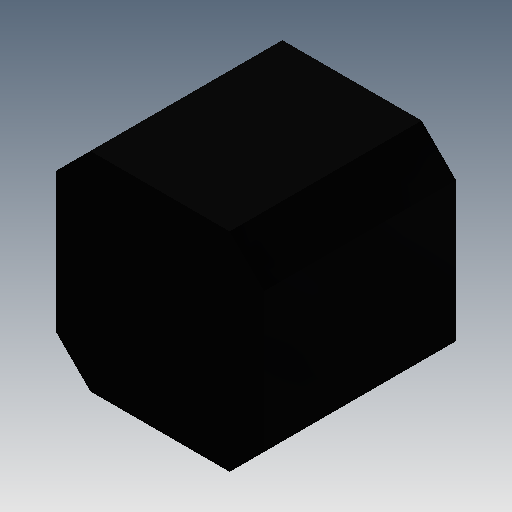
# Autodesk Inventor part: Nema 17 Body
Saved by Autodesk Inventor 2020.3 (Build 243373000, 373)
## iProperties
Created: 2015-09-21
Part Number: Nema 17 Body
Material: Aluminum 6061
Document SubType Name: Modeling
Designer: Dr Kreigar
Density: 2.7 g/cm^3
Appearance: Anodized - Black
Mass: 178.094 g
Surface Area: 93.4175 cm^2
Volume: 65.9607 cm^3
Author: Dr Kreigar
Autodesk Inventor part; units mm, degrees
ref_plane "YZ Plane" through (0, 0, 0) normal (1, 0, 0) x (0, 1, 0)
ref_plane "XZ Plane" through (0, 0, 0) normal (0, 1, 0) x (-1, 0, 0)
ref_plane "XY Plane" through (0, 0, 0) normal (0, 0, 1) x (1, 0, 0)
sketch "Sketch1" plane through (0, 0, 0) normal (0, 0, 1) x (1, 0, 0)
  line L0 (21.15, -14.1503) -> (21.15, 14.1503) construction
  line L1 (14.1503, 21.15) -> (21.15, 14.1503) construction
  line L2 (14.1503, 21.15) -> (-14.1503, 21.15) construction
  line L3 (-21.15, 14.1503) -> (-14.1503, 21.15) construction
  line L4 (-21.15, 14.1503) -> (-21.15, -14.1503) construction
  line L5 (-14.1503, -21.15) -> (-21.15, -14.1503) construction
  line L6 (-14.1503, -21.15) -> (14.1503, -21.15) construction
  line L7 (21.15, -14.1503) -> (14.1503, -21.15) construction
  line L8 (21.15, 14.1503) -> (14.1503, 21.15)
  line L9 (-14.1503, 21.15) -> (14.1503, 21.15)
  line L10 (-14.1503, 21.15) -> (-21.15, 14.1503)
  line L11 (-21.15, 14.1503) -> (-21.15, -14.1503)
  line L12 (-21.15, -14.1503) -> (-14.1503, -21.15)
  line L13 (-14.1503, -21.15) -> (14.1503, -21.15)
  line L14 (14.1503, -21.15) -> (21.15, -14.1503)
  line L15 (21.15, -14.1503) -> (21.15, 14.1503)
  point P0 (0, 0)
  constraints: 16 end point, 6 collinear
extrude "Extrusion1" add sketch "Sketch1" along normal blind 39
body "Solid1"
